disguise_v6 (Autodesk Fusion 360 design; units mm, degrees)
Autodesk Fusion 360 part; units mm, degrees
sketch "Esquisse1" plane through (0, 0, 0) normal (0, 0, 1) x (1, 0, 0) in component "Holder"
  circle A0 centre (0, 0) radius 3.25
  circle A1 centre (0, 0) radius 7.25
  line L0 (0, 7.25) -> (12.25, 7.25)
  line L1 (12.25, 7.25) -> (12.25, -7.25)
  line L2 (12.25, -7.25) -> (0, -7.25)
  line L3 (0, -7.25) -> (0, 7.25) construction
  dimension "d1" = 6.5
  dimension "d2" = 4
  dimension "d3" = 14.5
  dimension "d4" = 12.25
  constraint coincident A0.centre A1.centre
  constraint horizontal L0
  constraint vertical L1
  constraint horizontal L2
  constraint vertical L3
  constraint coincident A1 L0.start
  constraint midpoint A0.centre L3
  measures "d1" diameter of A0
  measures "d3" distance of L0.start L2.end
  measures "d4" distance of L0.start L0.end
extrude "Extrusion1" add sketch "Esquisse1" along normal blind 8 makes body 1 in component "Holder"
sketch "Esquisse3" plane through (0, -7.25, 0) normal (0, -1, 0) x (1, 0, 0) in component "Holder"
  line L0 (0, 0) -> (12.25, 0)
  line L1 (12.25, 0) -> (12.25, 8)
  line L2 (12.25, 8) -> (0, 8)
  line L3 (0, 8) -> (0, 0)
  circle A0 centre (8.25, 4) radius 4
  dimension "d14" = 8
  constraint tangent L2 A0
  constraint tangent L1 A0
  measures "d14" diameter of A0
pattern_circular "Réseau C2" count 2 over 90 about axis through (8.25, -7.25, 4) along (0, -1, 0) of bodies 1 makes body 2 in component "Holder"
sketch "Esquisse2" plane through (0, -7.25, 0) normal (0, -1, 0) x (1, 0, 0) in component "Holder"
  line L0 (0, 0) -> (12.25, 0)
  line L1 (12.25, 0) -> (12.25, 8)
  line L2 (12.25, 8) -> (0, 8)
  line L3 (0, 8) -> (0, 0)
  circle A0 centre (8.25, 4) radius 4
  circle A1 centre (8.25, 4) radius 2.55
  line L4 (0, 0) -> (-7.25, 0)
  line L5 (0, 0) -> (0, 8)
  line L6 (0, 8) -> (-7.25, 8)
  line L7 (0, 8) -> (0, 0)
  line L8 (-7.25, 8) -> (-7.25, 0)
  line L9 (8.25, 4) -> (12.25, 8) construction
  line L10 (8.25, 4) -> (8.4246, 8)
  line L11 (8.25, 4) -> (12.25, 4.1746)
  line L12 (8.25, 4) -> (0, 4) construction
  line L13 (5.1275, 6.5) -> (-7.25, 6.5)
  line L14 (-7.25, 6.5) -> (-7.25, 1.5)
  line L15 (-7.25, 1.5) -> (5.1275, 1.5)
  line L16 (5.1275, 1.5) -> (5.1275, 6.5) construction
  line L17 (5.75, -11.5) -> (10.75, -11.5)
  line L18 (5.75, 0.8775) -> (5.75, -11.5)
  line L19 (10.75, -11.5) -> (10.75, 0.8775)
  line L20 (12.25, -4.25) -> (12.25, -11.5)
  line L21 (12.25, -4.25) -> (4.25, -4.25)
  line L22 (4.25, -4.25) -> (4.25, -11.5)
  line L23 (4.25, -4.25) -> (12.25, -4.25)
  line L24 (12.25, -4.25) -> (12.25, 8)
  line L25 (12.25, 8) -> (4.25, 8)
  line L26 (4.25, 8) -> (4.25, -4.25)
  line L27 (4.25, -4.25) -> (12.25, -4.25)
  line L28 (4.25, -11.5) -> (12.25, -11.5)
  dimension "d7" = 8
  dimension "d8" = 5.1
  dimension "d21" = 85
  dimension "d22" = 5
  dimension "d24" = 90
  constraint tangent L2 A0
  constraint tangent L1 A0
  constraint concentric A0 A1
  constraint coincident A0.centre A1.centre
  constraint coincident L6.end L8.start
  constraint coincident L4.end L8.end
  constraint coincident L1.end L2.start
  constraint coincident L2 L10.end
  constraint coincident L1 L11.end
  constraint symmetric L9 L10 L11
  constraint midpoint L7 L12.end
  constraint horizontal L13
  constraint vertical L14
  constraint horizontal L15
  constraint vertical L16
  constraint coincident L8 L14.end
  constraint coincident A0 L13.start
  constraint symmetric L12 L13 L15
  constraint coincident L22.end L28.start
  constraint coincident L20.end L28.end
  measures "d7" diameter of A0
  measures "d8" diameter of A1
  measures "d21" angle of L10 L11
  measures "d22" distance of L13 L15
extrude "Extrusion4" cut sketch "Esquisse2" against normal through all contours L0 L3 L5 L7 L15 L26 | L3 L4 L5 L7 L8 L15 | L0 A0 L15 L18 L26 | L0 L18 L21 L23 L26 L27 | L18 L21 L22 L23 L27 L28 | L3 L5 L6 L7 L8 L13 | L2 L3 L5 L7 L13 L26 | L2 A0 L13 L25 L26 | L0 L1 A0 L19 L24 | L0 L19 L21 L23 L24 L27 | L19 L20 L21 L23 L27 L28 | L1 L2 A0 L10 L11 L24 L25 | A0 A1 L10 L11 | A1 L10 L11 | A1 L10 L11 picked at (8.7248, 7.4753) bodies 1 2 in component "Holder"
move_body "Déplacer2" bodies 1 2 to x (1, 0, 0) y (0, 0, 1) z (0, -1, 0) at (0, -0.75, 13.75) in component "Holder"
component "Holder" placed x (1, 0, 0) y (0, 1, 0) z (0, 0, 1) at (0, 0, 0)
equation "d3 = d1 + 2 * d2"
equation "d4 = d3 / 2 + 5 mm"
